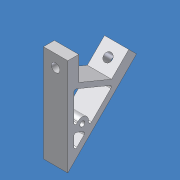
# Autodesk Inventor part: HBL45TS6hbl45ts6
Saved by Autodesk Inventor 2014 SP1 (Build 180222100, 222)
## iProperties
Category: PARTsolutions
Created: 2015-02-11
Part Number: HBL45TS6hbl45ts6
Catalog Web Link: www.cadenas.de
Description: HBL45TS6, HBL45TD6, HBL135TS6, HBL135TD6 - Brackets with Angle 45/135 Deg.
Document SubType Name: Modeling
Designer: PARTsolutions
Material: Generic
Density: 1 g/cm^3
Appearance: RGB(192,192,192)
NB: HBL45TS6hbl45ts6
NN: HBL45TS6, HBL45TD6, HBL135TS6, HBL135TD6
NT: Brackets with Angle 45/135 Deg.
NBSYN: $PN.hbl45ts6
LINA: HBL45TS6hbl45ts6
PN: HBL45TS6
TP: HBL45TS6
MAT: JIS-A6N01SS-T5
ST: Anodizing
TYPE: HBL45TS6
FEAT: Brackets with Angle 45 Deg.
SLOT: Slot Width 8 Frame
MASS: 58
AB: CBM6-15
NOB: 2
AN: HNTT6-6
NON: 2
AL: 1176
W: 20
DIA: 7.0
ALT1OPT: '','w/o C (Mounting Holes for Cover)','-C','with C (Mounting Holes for Cover)'
VER: 5
DIS: 0.000
VERS: 5.000
KT: 5
SUPPLIER: Misumi
ARTICLENO: HBL45TS6hbl45ts6
BOMINFO: HBL45TS6hbl45ts6
CREATOR: CADENAS GmbH
PSOL_IDENT_0: {\\10.0.0.236\data_v8\23d-libs\misumi\metric\38_al_extrusions_blackets\6\hbl45ts6.prj},218 {VTYP=3D}
PSOL_IDENT_1: ,{NB=HBL45TS6hbl45ts6},{LINA=HBL45TS6hbl45ts6},{NN=HBL45TS6, HBL45TD6, HBL135TS6, HBL135TD6},{DATE=1
PSOL_IDENT_2: 9.11.2014 02:28:17},{GEOMDATE=12.03.2009 12:55:00},{VERSION=},{LINEID=260},{LINESUBID=-1},{WBVAR=ALT
PSOL_IDENT_3: 1,ALT3}  {NB=HBL45TS6hbl45ts6},{LINA=HBL45TS6hbl45ts6},{KT=5},{PN=HBL45TS6},{TP=HBL45TS6},{MAT=JIS-A
PSOL_IDENT_4: 6N01SS-T5},{ST=Anodizing},{TYPE=HBL45TS6},{FEAT=Brackets with Angle 45 Deg.},{SLOT=Slot Width 8 Fram
PSOL_IDENT_5: e},{ALT1=},{ALT3=},{MASS=58},{AB=CBM6-15},{NOB=2},{AN=HNTT6-6},{NON=2},{AL=1176},{W=20},{DIA=7.0},{A
PSOL_IDENT_6: LT1OPT='','w/o C (Mounting Holes for Cover)','-C','with C (Mounting Holes for Cover)'},{VER=5},{DIS=
PSOL_IDENT_7: 0.000},{VERS=5.000}
Title: HBL45TS6hbl45ts6
Author: Cadenas PARTsolutions
Comments: Brackets with Angle 45/135 Deg.
Autodesk Inventor part; units mm, degrees
sketch "Sketch_1" plane through (0, 0, 0) normal (1, 0, 0) x (0, 1, 0)
  line L0 (0, 80) -> (0, 0)
  line L1 (0, 0) -> (56.5685, 56.5685)
  line L2 (56.5685, 56.5685) -> (50.2046, 62.9325)
  line L3 (50.2046, 62.9325) -> (36.0624, 48.7904)
  line L4 (36.0624, 48.7904) -> (9, 60)
  line L5 (9, 60) -> (9, 80)
  line L6 (9, 80) -> (0, 80)
  arc A0 (6.8931, 25.3806) -> (5, 23.933) centre (6.5, 23.933) ccw
  line L7 (5, 23.933) -> (5, 15.6924)
  arc A1 (5, 15.6924) -> (7.5607, 14.6317) centre (6.5, 15.6924) ccw
  line L8 (7.5607, 14.6317) -> (13.3877, 20.4587)
  arc A2 (13.3877, 20.4587) -> (13.0726, 22.821) centre (12.327, 21.5194) ccw
  arc A3 (13.0726, 22.821) -> (6.8931, 25.3806) centre (0, 0) ccw
  circle A4 centre (12, 28.9706) radius 2.1
  arc A5 (7.074, 56.4682) -> (5, 55.0824) centre (6.5, 55.0824) ccw
  line L9 (5, 55.0824) -> (5, 32.7559)
  arc A6 (5, 32.7559) -> (7.5929, 31.7285) centre (6.5, 32.7559) ccw
  line L10 (7.5929, 31.7285) -> (8.2843, 32.4639)
  arc A7 (17.0976, 28.8133) -> (8.2843, 32.4639) centre (12, 28.9706) ccw
  line L11 (17.0976, 28.8133) -> (17.0665, 27.8044)
  arc A8 (17.0665, 27.8044) -> (19.6264, 26.6975) centre (18.5657, 27.7581) ccw
  line L12 (19.6264, 26.6975) -> (35.4136, 42.4847)
  arc A9 (35.4136, 42.4847) -> (34.927, 44.9311) centre (34.3529, 43.5453) ccw
  line L13 (34.927, 44.9311) -> (7.074, 56.4682)
  constraints: 28 end point, 18 point on circle, 10 centre point
extrude "Extrusion1" add sketch "Sketch_1" along normal mid plane 20
sketch "Sketch_2" plane through (-10, 50.2046, 62.9325) normal (0, -0.7071, 0.7071) x (1, 0, 0)
  circle A0 centre (10, -10) radius 3.5
  constraints: 1 centre point
extrude "Extrusion2" cut sketch "Sketch_2" against normal blind 9
sketch "Sketch_3" plane through (0, 0, 0) normal (0, 1, 0) x (-1, 0, 0)
  circle A0 centre (0, 70) radius 3.5
  constraints: 1 centre point
extrude "Extrusion3" cut sketch "Sketch_3" along normal blind 9
ref_plane "bracket_to_dummy_XY" through (0, 0, 0) normal (0, 1, 0) x (1, 0, 0)
ref_plane "bracket_to_dummy_YZ" through (0, 0, 0) normal (1, 0, 0) x (0, 0, -1)
ref_plane "bracket_to_dummy_ZX" through (0, 0, 0) normal (0, 0, -1) x (0, 1, 0)
ref_plane "1_to_bolt_XY" through (0, 9, 70) normal (0, 1, 0) x (1, 0, 0)
ref_plane "1_to_bolt_YZ" through (0, 9, 70) normal (1, 0, 0) x (0, 0, -1)
ref_plane "1_to_bolt_ZX" through (0, 9, 70) normal (0, 0, -1) x (0, 1, 0)
ref_plane "2_to_bolt_XY" through (0, 43.1335, 55.8614) normal (0, -0.7071, 0.7071) x (0, 0.7071, 0.7071)
ref_plane "2_to_bolt_YZ" through (0, 43.1335, 55.8614) normal (0, 0.7071, 0.7071) x (-1, 0, 0)
ref_plane "2_to_bolt_ZX" through (0, 43.1335, 55.8614) normal (-1, 0, 0) x (0, -0.7071, 0.7071)
ref_plane "3_to_bolt_XY" through (0, 9, 70) normal (0, 1, 0) x (0, 0, -1)
ref_plane "3_to_bolt_YZ" through (0, 9, 70) normal (0, 0, -1) x (-1, 0, 0)
ref_plane "3_to_bolt_ZX" through (0, 9, 70) normal (-1, 0, 0) x (0, 1, 0)
ref_plane "4_to_bolt_XY" through (30, 9, 70) normal (0, 1, 0) x (0, 0, -1)
ref_plane "4_to_bolt_YZ" through (30, 9, 70) normal (0, 0, -1) x (-1, 0, 0)
ref_plane "4_to_bolt_ZX" through (30, 9, 70) normal (-1, 0, 0) x (0, 1, 0)
ref_plane "5_to_bolt_XY" through (30, 43.1335, 55.8614) normal (0, -0.7071, 0.7071) x (0, 0.7071, 0.7071)
ref_plane "5_to_bolt_YZ" through (30, 43.1335, 55.8614) normal (0, 0.7071, 0.7071) x (-1, 0, 0)
ref_plane "5_to_bolt_ZX" through (30, 43.1335, 55.8614) normal (-1, 0, 0) x (0, -0.7071, 0.7071)
body "Solid1"
